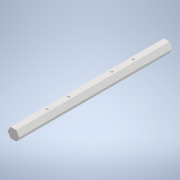
# Autodesk Inventor part: Eje1
Saved by Autodesk Inventor 2022 (Build 260153000, 153)
## iProperties
Created: 2022-02-21
Part Number: Eje1
Material: Generic
Document SubType Name: Modeling
Designer: katha
Density: 1 g/cm^3
Appearance: Default
Author: katha
Autodesk Inventor part; units mm, degrees
ref_plane "YZ Plane" through (0, 0, 0) normal (1, 0, 0) x (0, 1, 0)
ref_plane "XZ Plane" through (0, 0, 0) normal (0, 1, 0) x (-1, 0, 0)
ref_plane "XY Plane" through (0, 0, 0) normal (0, 0, 1) x (1, 0, 0)
sketch "Sketch1" plane through (0, 0, 0) normal (0, 0, 1) x (1, 0, 0)
  line L0 (-92.355, 44.9365) -> (-95.7014, 44.9365) projected
  line L1 (-90.6818, 47.8346) -> (-92.355, 44.9365) projected
  line L2 (-92.355, 50.7327) -> (-90.6818, 47.8346) projected
  line L3 (-95.7014, 50.7327) -> (-92.355, 50.7327) projected
  line L4 (-97.3746, 47.8346) -> (-95.7014, 50.7327) projected
  line L5 (-95.7014, 44.9365) -> (-97.3746, 47.8346) projected
  line L6 (-95.7014, 50.7327) -> (-92.355, 44.9365) construction
  line L7 (-95.7014, 44.9365) -> (-92.355, 50.7327) construction
  line L8 (-97.3746, 47.8346) -> (-90.6818, 47.8346) construction
  line L9 (-94.0282, 47.8346) -> (-91.0282, 47.8346)
  circle A0 centre (-94.0282, 47.8346) radius 3.3464 construction
  line L10 (-94.0282, 47.8346) -> (-92.5282, 50.4327)
  line L11 (-94.0282, 47.8346) -> (-95.5282, 50.4327)
  line L12 (-94.0282, 47.8346) -> (-97.0282, 47.8346)
  line L13 (-94.0282, 47.8346) -> (-95.5282, 45.2365)
  line L14 (-94.0282, 47.8346) -> (-92.5282, 45.2365)
  line L15 (-95.5282, 50.4327) -> (-92.5282, 50.4327)
  line L16 (-92.5282, 50.4327) -> (-91.0282, 47.8346)
  line L17 (-91.0282, 47.8346) -> (-92.5282, 45.2365)
  line L18 (-92.5282, 45.2365) -> (-95.5282, 45.2365)
  line L19 (-95.5282, 45.2365) -> (-97.0282, 47.8346)
  line L20 (-97.0282, 47.8346) -> (-95.5282, 50.4327)
  point P0 (0, 0)
  dimension "d0" = 3
  dimension "d4" = 360
  constraints: 30 end point, 3 parallel, 2 horizontal, 1 coincident, 1 midpoint, 1 point on line, 22 other
  measures "d0" distance of L9.start L9.end
extrude "Extrusion2" add sketch "Sketch1" along normal blind 80 contours L10 L16 L9 | L11 L15 L10 | L12 L20 L11 | L13 L19 L12 | L14 L18 L13 | L9 L17 L14
sketch "Sketch2" plane through (-95.5282, 50.4327, 0) normal (0, 1, 0) x (1, 0, 0)
  circle A0 centre (1.5, -17.5) radius 0.625 projected
  circle A1 centre (1.5, -28.7) radius 0.625 projected
  circle A2 centre (1.5, -51.3) radius 0.625 projected
  circle A3 centre (1.5, -62.5) radius 0.625 projected
  point P0 (95.5282, 0)
extrude "Extrusion3" cut sketch "Sketch2" against normal blind 10
body "Solid2"
